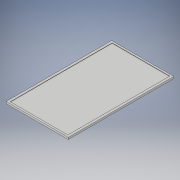
# Autodesk Inventor part: LCD Screen
Saved by Autodesk Inventor 2017 (Build 210142000, 142)
## iProperties
Created: 2019-02-16
Part Number: LCD Screen
Material: Generic
Document SubType Name: Modeling
Designer: Mitch
Density: 1 g/cm^3
Appearance: Default
Author: Mitch
Autodesk Inventor part; units mm, degrees
ref_plane "YZ Plane" through (0, 0, 0) normal (1, 0, 0) x (0, 1, 0)
ref_plane "XZ Plane" through (0, 0, 0) normal (0, 1, 0) x (-1, 0, 0)
ref_plane "XY Plane" through (0, 0, 0) normal (0, 0, 1) x (1, 0, 0)
sketch "Sketch1" plane through (0, 0, 0) normal (0, 1, 0) x (-1, 0, 0)
  line L0 (0, 0) -> (296.8625, 0)
  line L1 (296.8625, 0) -> (296.8625, -525.4625)
  line L2 (296.8625, -525.4625) -> (0, -525.4625)
  line L3 (0, -525.4625) -> (0, 0)
  line L4 (308.7687, 9.525) -> (-11.9063, 9.525)
  line L5 (-11.9063, 9.525) -> (-11.9062, -534.9875)
  line L6 (-11.9062, -534.9875) -> (308.7688, -534.9875)
  line L7 (308.7688, -534.9875) -> (308.7687, 9.525)
  dimension "d0" = 296.8625
  dimension "d1" = 525.4625
  dimension "d4" = 11.9062
  dimension "d5" = 11.9062
  dimension "d6" = 9.525
  dimension "d7" = 9.525
  constraints: 16 end point, 4 parallel, 2 horizontal, 2 perpendicular
  measures "d0" distance of L1.end L2.end
  measures "d1" distance of L0.end L1.end
  measures "d4" distance between parallel lines of L1 L7
  measures "d5" distance between parallel lines of L3 L5
  measures "d6" distance between parallel lines of L0 L4
  measures "d7" distance between parallel lines of L2 L6
extrude "Extrusion1" add sketch "Sketch1" along normal blind 9.7282 contours L0 L1 L2 L3 | L7 L6 L5 L4
sketch "Sketch2" plane through (0, 9.7282, 0) normal (0, 1, 0) x (1, 0, 0)
  line L0 (-296.8562, 0) -> (-0.0063, 0)
  line L1 (-0.0063, 0) -> (-0.0064, 525.4625)
  line L2 (-0.0064, 525.4625) -> (-296.8562, 525.4625)
  line L3 (-296.8562, 525.4625) -> (-296.8562, 0)
  line L4 (-308.7688, 534.9875) -> (-308.7687, -9.525) projected
  line L5 (-308.7687, -9.525) -> (11.9063, -9.525) projected
  line L6 (11.9062, 534.9875) -> (-308.7688, 534.9875) projected
  line L7 (11.9063, -9.525) -> (11.9062, 534.9875) projected
  point P0 (0, 0)
  dimension "d10" = 11.9126
  dimension "d11" = 9.525
  dimension "d12" = 9.525
  dimension "d13" = 11.9126
  constraints: 8 end point, 2 parallel, 1 horizontal, 1 perpendicular
  measures "d10" distance between parallel lines of L4 L3
  measures "d11" distance between parallel lines of L5 L0
  measures "d12" distance between parallel lines of L6 L2
  measures "d13" distance between parallel lines of L7 L1
extrude "Extrusion2" cut sketch "Sketch2" against normal blind 1.5875 contours L3 L2 L1 L0
body "Solid1"
